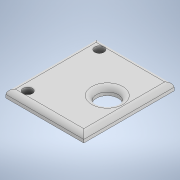
# Autodesk Inventor part: Деталь5
Saved by Autodesk Inventor 2020 (Build 240168000, 168)
## iProperties
Created: 2021-07-25
Part Number: Деталь5
Material: Типовые
Document SubType Name: Modeling
Designer: PC
Density: 1 g/cm^3
Appearance: По умолчанию
Author: PC
Autodesk Inventor part; units mm, degrees
ref_plane "YZ Plane" through (0, 0, 0) normal (1, 0, 0) x (0, 1, 0)
ref_plane "XZ Plane" through (0, 0, 0) normal (0, 1, 0) x (-1, 0, 0)
ref_plane "XY Plane" through (0, 0, 0) normal (0, 0, 1) x (1, 0, 0)
sketch "Эскиз1" plane through (0, 0, 0) normal (0, 1, 0) x (-1, 0, 0)
  line L0 (6.8605, 9.6174) -> (-18.1395, 9.6174)
  line L1 (-18.1395, 9.6174) -> (-18.1395, -19.3826)
  line L2 (-18.1395, -19.3826) -> (6.8605, -19.3826)
  line L3 (6.8605, -19.3826) -> (6.8605, 9.6174)
  circle A0 centre (2.8605, 6.6174) radius 1.5
  circle A1 centre (2.8605, -16.3826) radius 1.5
  circle A2 centre (-11.2073, -4.8826) radius 3.5
  point P0 (0, 0)
  dimension "d0" = 3
  dimension "d1" = 3
  dimension "d2" = 23
  dimension "d3" = 3
  dimension "d4" = 3
  dimension "d5" = 25
  dimension "d6" = 4
  dimension "d7" = 7
  constraints: 8 end point, 3 centre point, 2 parallel, 1 horizontal, 1 perpendicular
  measures "d0" diameter of A0
  measures "d1" diameter of A1
  measures "d2" distance of A1.centre A0.centre
  measures "d3" distance from line of A0.centre L0
  measures "d4" distance from line of L2 A1.centre
  measures "d5" distance of L1.end L2.end
  measures "d6" distance from line of L3 A0.centre
  measures "d7" diameter of A2
extrude "Выдавливание1" add sketch "Эскиз1" along normal blind 2.5
fillet "Сопряжение1" radius 1.5 1 edges at (14.7073, 2.5, -4.8826)
fillet "Сопряжение2" radius 1.5 4 edges at (5.6395, 2.5, 9.6174) (18.1395, 2.5, -4.8826) (5.6395, 2.5, -19.3826) (-6.8605, 2.5, -4.8826)
